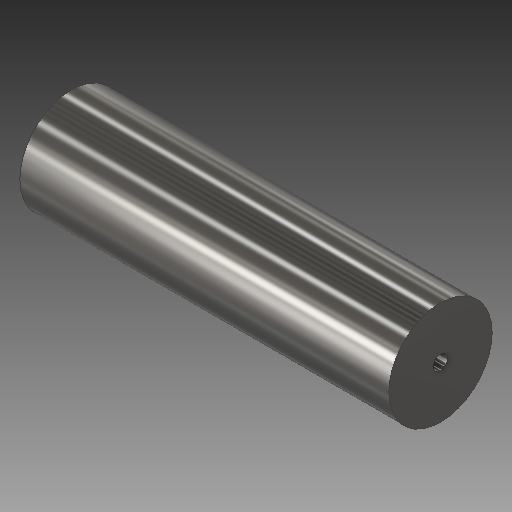
# Autodesk Inventor part: BearingCJE
Saved by Autodesk Inventor 2018 (Build 220112000, 112)
## iProperties
Created: 2018-02-03
Part Number: BearingCJE
Material: Steel, Alloy
Document SubType Name: Modeling
Designer: textboox5
Density: 7.73 g/cm^3
Appearance: Polished - Small Pyramid Knurl
Author: textboox5
Autodesk Inventor part; units mm, degrees
ref_plane "YZ Plane" through (0, 0, 0) normal (1, 0, 0) x (0, 1, 0)
ref_plane "XZ Plane" through (0, 0, 0) normal (0, 1, 0) x (-1, 0, 0)
ref_plane "XY Plane" through (0, 0, 0) normal (0, 0, 1) x (1, 0, 0)
sketch "Sketch1" plane through (0, 0, 0) normal (0, 0, 1) x (1, 0, 0)
  line L0 (-939.8, 355.6) -> (-939.8, 50.8)
  line L1 (-939.8, 50.8) -> (-736.6, 50.8)
  line L2 (-736.6, 50.8) -> (-736.6, 0)
  line L3 (-736.6, 0) -> (1397, 0)
  line L4 (1397, 0) -> (1397, 50.8)
  line L5 (1397, 50.8) -> (1600.2, 50.8)
  line L6 (1600.2, 50.8) -> (1600.2, 355.6)
  line L7 (1600.2, 355.6) -> (-939.8, 355.6)
  line L8 (330.2, 355.6) -> (330.2, 0) construction
  line L9 (1397, -50.8) -> (1397, 50.8) construction
  line L10 (-736.6, -50.8) -> (-736.6, 50.8) construction
  line L11 (1397, 50.8) -> (1651, 50.8) construction
  line L12 (1651, -12.7187) -> (1651, 85.4194) construction
  line L13 (-737.4384, -17394.9442) -> (1396.1616, -17394.9442)
  point P0 (-736.6, 0)
  dimension "d1" = 711.2
  dimension "d5" = 50.8
  constraints: 22 end point, 7 perpendicular, 3 midpoint, 2 collinear, 2 horizontal, 2 vertical, 1 point on line, 4 other
  measures "d1" diameter of L7 L3
  measures "d5" distance between parallel lines of L6 L12
revolve "Revolution1" add sketch "Sketch1" angle 360 about axis through (-736.6, 0, 0) along (1, 0, 0)
body "Solid1"
